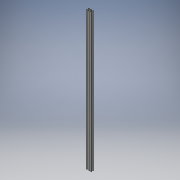
# Autodesk Inventor part: PERFIL_ESTRUTURAL_20X40_MESA
Saved by Autodesk Inventor 2018 (Build 220112000, 112)
## iProperties
Created: 2018-10-25
Part Number: PERFIL_ESTRUTURAL_20X40_MESA
Material: Genérico
Document SubType Name: Modeling
Designer: Georgines
Density: 1 g/cm^3
Appearance: Padrão
Author: Georgines
Autodesk Inventor part; units mm, degrees
ref_plane "YZ Plane" through (0, 0, 0) normal (1, 0, 0) x (0, 1, 0)
ref_plane "XZ Plane" through (0, 0, 0) normal (0, 1, 0) x (-1, 0, 0)
ref_plane "XY Plane" through (0, 0, 0) normal (0, 0, 1) x (1, 0, 0)
sketch "Esboço1" plane through (0, 0, 0) normal (0, 0, 1) x (1, 0, 0)
  arc A0 (19, -10) -> (20, -9) centre (19, -9) ccw
  line L0 (20, -4.8) -> (20, -9)
  line L1 (18.2, -3) -> (20, -4.8)
  line L2 (18.2, -5.5) -> (18.2, -3)
  line L3 (16.5607, -5.5) -> (18.2, -5.5)
  line L4 (14, -2.9393) -> (16.5607, -5.5)
  line L5 (14, -0.3) -> (14, -2.9393)
  line L6 (13.7, 0) -> (14, -0.3)
  line L7 (14, 0.3) -> (13.7, 0)
  line L8 (14, 2.9393) -> (14, 0.3)
  line L9 (16.5607, 5.5) -> (14, 2.9393)
  line L10 (18.2, 5.5) -> (16.5607, 5.5)
  line L11 (18.2, 3) -> (18.2, 5.5)
  line L12 (20, 4.8) -> (18.2, 3)
  line L13 (20, 9) -> (20, 4.8)
  arc A1 (20, 9) -> (19, 10) centre (19, 9) ccw
  line L14 (14.8, 10) -> (19, 10)
  line L15 (13, 8.2) -> (14.8, 10)
  line L16 (15.5, 8.2) -> (13, 8.2)
  line L17 (15.5, 6.5607) -> (15.5, 8.2)
  line L18 (12.9393, 4) -> (15.5, 6.5607)
  line L19 (10.3, 4) -> (12.9393, 4)
  line L20 (10, 3.7) -> (10.3, 4)
  line L21 (9.7, 4) -> (10, 3.7)
  line L22 (7.0607, 4) -> (9.7, 4)
  line L23 (4.5, 6.5607) -> (7.0607, 4)
  line L24 (4.5, 8.2) -> (4.5, 6.5607)
  line L25 (7, 8.2) -> (4.5, 8.2)
  line L26 (5.2, 10) -> (7, 8.2)
  line L27 (-5.2, 10) -> (5.2, 10)
  line L28 (-7, 8.2) -> (-5.2, 10)
  line L29 (-4.5, 8.2) -> (-7, 8.2)
  line L30 (-4.5, 6.5607) -> (-4.5, 8.2)
  line L31 (-7.0607, 4) -> (-4.5, 6.5607)
  line L32 (-9.7, 4) -> (-7.0607, 4)
  line L33 (-10, 3.7) -> (-9.7, 4)
  line L34 (-10.3, 4) -> (-10, 3.7)
  line L35 (-12.9393, 4) -> (-10.3, 4)
  line L36 (-15.5, 6.5607) -> (-12.9393, 4)
  line L37 (-15.5, 8.2) -> (-15.5, 6.5607)
  line L38 (-13, 8.2) -> (-15.5, 8.2)
  line L39 (-14.8, 10) -> (-13, 8.2)
  line L40 (-19, 10) -> (-14.8, 10)
  arc A2 (-19, 10) -> (-20, 9) centre (-19, 9) ccw
  line L41 (-20, 4.8) -> (-20, 9)
  line L42 (-18.2, 3) -> (-20, 4.8)
  line L43 (-18.2, 5.5) -> (-18.2, 3)
  line L44 (-16.5607, 5.5) -> (-18.2, 5.5)
  line L45 (-14, 2.9393) -> (-16.5607, 5.5)
  line L46 (-14, 0.3) -> (-14, 2.9393)
  line L47 (-13.7, 0) -> (-14, 0.3)
  line L48 (-14, -0.3) -> (-13.7, 0)
  line L49 (-14, -2.9393) -> (-14, -0.3)
  line L50 (-16.5607, -5.5) -> (-14, -2.9393)
  line L51 (-18.2, -5.5) -> (-16.5607, -5.5)
  line L52 (-18.2, -3) -> (-18.2, -5.5)
  line L53 (-20, -4.8) -> (-18.2, -3)
  line L54 (-20, -9) -> (-20, -4.8)
  arc A3 (-20, -9) -> (-19, -10) centre (-19, -9) ccw
  line L55 (-14.8, -10) -> (-19, -10)
  line L56 (-13, -8.2) -> (-14.8, -10)
  line L57 (-15.5, -8.2) -> (-13, -8.2)
  line L58 (-15.5, -6.5607) -> (-15.5, -8.2)
  line L59 (-12.9393, -4) -> (-15.5, -6.5607)
  line L60 (-10.3, -4) -> (-12.9393, -4)
  line L61 (-10, -3.7) -> (-10.3, -4)
  line L62 (-9.7, -4) -> (-10, -3.7)
  line L63 (-7.0607, -4) -> (-9.7, -4)
  line L64 (-4.5, -6.5607) -> (-7.0607, -4)
  line L65 (-4.5, -8.2) -> (-4.5, -6.5607)
  line L66 (-7, -8.2) -> (-4.5, -8.2)
  line L67 (-5.2, -10) -> (-7, -8.2)
  line L68 (5.2, -10) -> (-5.2, -10)
  line L69 (7, -8.2) -> (5.2, -10)
  line L70 (4.5, -8.2) -> (7, -8.2)
  line L71 (4.5, -6.5607) -> (4.5, -8.2)
  line L72 (7.0607, -4) -> (4.5, -6.5607)
  line L73 (9.7, -4) -> (7.0607, -4)
  line L74 (10, -3.7) -> (9.7, -4)
  line L75 (10.3, -4) -> (10, -3.7)
  line L76 (12.9393, -4) -> (10.3, -4)
  line L77 (15.5, -6.5607) -> (12.9393, -4)
  line L78 (15.5, -8.2) -> (15.5, -6.5607)
  line L79 (13, -8.2) -> (15.5, -8.2)
  line L80 (14.8, -10) -> (13, -8.2)
  line L81 (19, -10) -> (14.8, -10)
  line L82 (-2.7, 8.2) -> (2.7, 8.2)
  line L83 (2.7, 8.2) -> (2.7, 6.2393)
  line L84 (2.7, 6.2393) -> (6, 2.9393)
  line L85 (6, 2.9393) -> (6, -2.9393)
  line L86 (6, -2.9393) -> (2.7, -6.2393)
  line L87 (2.7, -6.2393) -> (2.7, -8.2)
  line L88 (2.7, -8.2) -> (-2.7, -8.2)
  line L89 (-2.7, -8.2) -> (-2.7, -6.2393)
  line L90 (-2.7, -6.2393) -> (-6, -2.9393)
  line L91 (-6, -2.9393) -> (-6, 2.9393)
  line L92 (-6, 2.9393) -> (-2.7, 6.2393)
  line L93 (-2.7, 6.2393) -> (-2.7, 8.2)
  circle A4 centre (10, 0) radius 2.5
  circle A5 centre (-10, 0) radius 2.5
  point P0 (0, 0)
  point P1 (0, 0)
  constraints: 188 end point, 8 point on circle, 6 centre point
extrude "Extrusão1" add sketch "Esboço1" along normal blind 1054
